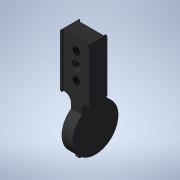
# Autodesk Inventor part: 1310164 DHRS-32-A---(Griff)
Saved by Autodesk Inventor 2025.1 (Build 291241000, 241)
## iProperties
Category: PARTsolutions
Company: FESTO
Created: 2025-06-16
Part Number: 1310164 DHRS-32-A---(Griff)
Material: Generic
Catalog Web Link: www.cadenas.de
Description: DHRS---(Griff)-Handle
Vendor: FESTO
Document SubType Name: Modeling
Designer: psAdmin
Manufacturer: FESTO
Mass: 6.83558 g
Surface Area: 36.2537 cm^2
Volume: 6.83558 cm^3
Density: 1 g/cm^3
Appearance: PSOLRGB-175-175-175
PSOL_IDENT_0: {$CADENAS_DATA/23d-libs/festo/parts/d/dhrs/parts/dhrs_griff.prj},202 {VTYP=3D},{NB=1310164 DHRS-32-A
PSOL_IDENT_1: ---(Griff)},{LINA=1310164 DHRS-32-A---(Griff)},{NN=DHRS---(Griff)},{DATE=04.06.2025 19:34:44},{GEOMD
PSOL_IDENT_2: ATE=22.08.2023 11:13:58},{VERSION=},{LINEID=60},{WBVAR=},{WBNUMERIC=}  {NB=1310164 DHRS-32-A---(Grif
PSOL_IDENT_3: f)},{LINA=1310164 DHRS-32-A---(Griff)},{KT=DUMMY},{TNR=1310164},{TYP=DHRS-32-A},{GR=32}
NB: 1310164 DHRS-32-A---(Griff)
NN: DHRS---(Griff)
NT: Handle
NBSYN: $TNR. $TYP.---(Griff)
LINA: 1310164 DHRS-32-A---(Griff)
CATALOG: Festo
TNR: 1310164
TYP: DHRS-32-A
GR: 32
SUPPLIER: FESTO
ARTICLENO: 1310164 DHRS-32-A---(Griff)
BOMINFO: 1310164 DHRS-32-A---(Griff)
CREATOR: CADENAS GmbH
Title: 1310164 DHRS-32-A---(Griff)
Author: Cadenas PARTsolutions
Comments: Handle
Autodesk Inventor part; units mm, degrees
sketch "Sketch_1" plane through (0, 0, 0) normal (1, 0, 0) x (0, 1, 0)
  arc A0 (10.1247, 7.5) -> (12.3488, -2.5033) centre (0, 0) ccw
  arc A1 (14.799, -0.5) -> (12.3488, -2.5033) centre (14.799, -3) ccw
  line L0 (14.799, -0.5) -> (46, -0.5)
  line L1 (46, -0.5) -> (46, 7.5)
  line L2 (46, 7.5) -> (10.1247, 7.5)
  constraints: 6 end point, 4 point on circle, 2 centre point
extrude "Extrusion1" add sketch "Sketch_1" along normal mid plane 14
sketch "Sketch_2" plane through (0, 0, 0) normal (0, 0, 1) x (1, 0, 0)
  line L0 (-7, -24.7) -> (7, -24.7)
  line L1 (7, -24.7) -> (7, 16.5)
  line L2 (7, 16.5) -> (6.5, 16.5)
  arc A0 (6.5, 16.5) -> (3, 13) centre (6.5, 13) ccw
  line L3 (3, 13) -> (3, -21.7)
  line L4 (3, -21.7) -> (-3, -21.7)
  line L5 (-3, -21.7) -> (-3, 13)
  arc A1 (-3, 13) -> (-6.5, 16.5) centre (-6.5, 13) ccw
  line L6 (-6.5, 16.5) -> (-7, 16.5)
  line L7 (-7, 16.5) -> (-7, -24.7)
  constraints: 16 end point, 4 point on circle, 2 centre point
extrude "Extrusion2" cut sketch "Sketch_2" along normal mid plane 30
sketch "Sketch_3" plane through (0, 0, 8.5) normal (0, 0, 1) x (1, 0, 0)
  line L0 (7, 16.5) -> (7.5, 16.5)
  line L1 (7.5, 16.5) -> (8, 17)
  line L2 (8, 17) -> (8, 45.5)
  line L3 (8, 45.5) -> (7.5, 46)
  line L4 (7.5, 46) -> (7, 46)
  line L5 (7, 46) -> (7, 16.5)
  constraints: 12 end point
extrude "Extrusion3" add sketch "Sketch_3" against normal blind 10
sketch "Sketch_4" plane through (0, 0, 8.5) normal (0, 0, 1) x (1, 0, 0)
  line L0 (-8, 17) -> (-7.5, 16.5)
  line L1 (-7.5, 16.5) -> (-7, 16.5)
  line L2 (-7, 16.5) -> (-7, 46)
  line L3 (-7, 46) -> (-7.5, 46)
  line L4 (-7.5, 46) -> (-8, 45.5)
  line L5 (-8, 45.5) -> (-8, 17)
  constraints: 12 end point
extrude "Extrusion4" add sketch "Sketch_4" against normal blind 10
sketch "Sketch_5" plane through (0, 0, 0) normal (1, 0, 0) x (0, 1, 0)
  line L0 (32, -0.5) -> (32, 7.5)
  line L1 (32, 7.5) -> (34.5, 7.5)
  line L2 (34.5, 7.5) -> (34, 7)
  line L3 (34, 7) -> (34, 0)
  line L4 (34, 0) -> (34.5, -0.5)
  line L5 (34.5, -0.5) -> (32, -0.5)
  line L6 (32, -0.5) -> (32, 7.5)
  constraints: 14 end point
revolve "Revolution1" cut sketch "Sketch_5" angle 360 about axis through (0, 32, -0.5) along (0, 0, -1)
sketch "Sketch6" plane through (-3, 10.1247, 7.5) normal (0, 0, 1) x (1, 0, 0)
  point P0 (3, 14.8753)
hole "Hole1" at (0, 25, 7.5) direction (0, 0, -1) diameter 4.134 depth 8 thread size "M5x0.8" class "6H" standard "ISO Metric profile"
sketch "Sketch7" plane through (-3, 10.1247, 7.5) normal (0, 0, 1) x (1, 0, 0)
  point P0 (3, 28.8753)
hole "Hole2" at (0, 39, 7.5) direction (0, 0, -1) diameter 4.134 depth 8 thread size "M5x0.8" class "6H" standard "ISO Metric profile"
sketch "Sketch_9" plane through (0, 0, 0) normal (1, 0, 0) x (0, 1, 0)
  arc A0 (-11.5335, 7.2069) -> (-12.1177, 6.1743) centre (0, 0) ccw
  line L0 (-12.1177, 6.1743) -> (0, 0)
  line L1 (0, 0) -> (-11.5335, 7.2069)
  constraints: 4 end point, 2 point on circle, 1 centre point
extrude "Extrusion5" add sketch "Sketch_9" along normal mid plane 2
ref_plane "GRIFF_XY" through (0, 0, 0) normal (1, 0, 0) x (0, 0, -1)
ref_plane "GRIFF_YZ" through (0, 0, 0) normal (0, 0, -1) x (0, 1, 0)
ref_plane "GRIFF_ZX" through (0, 0, 0) normal (0, 1, 0) x (1, 0, 0)
body "Solid1"
